cactusholder (Autodesk Fusion 360 design; units mm, degrees)
Autodesk Fusion 360 part; units mm, degrees
sketch "Sketch1" plane through (0, 0, 0) normal (0, 0, 1) x (1, 0, 0)
  circle A0 centre (0, 0) radius 37.5
  circle A1 centre (41.1956, 26.2031) radius 5
  spline S0 degree 5 poles (-34.1248, 15.5483) (-34.2892, 15.7362) (-35.0019, 16.448) (-36.6305, 17.4055) (-39.8225, 17.9751) (-44.8611, 17.5874) (-50.2206, 16.9014) (-53.5274, 17.4394) (-53.931, 20.0284) (-51.715, 24.3952) (-48.5491, 28.6137) (-45.8719, 31.6881) (-44.0593, 33.5751) (-43.1537, 34.4673) (-42.248, 35.3596) (-40.4379, 37.0417) (-37.7714, 39.1944) (-34.3544, 41.1861) (-30.0177, 42.3086) (-25.2467, 42.4584) (-19.8767, 42.1915) (-14.3394, 42.0733) (-9.6412, 42.5862) (-6.8287, 44.1058) (-6.6326, 46.8627) (-8.9316, 50.901) (-12.8621, 56.0874) (-17.1953, 62.1454) (-20.6408, 68.6812) (-22.1573, 75.2143) (-21.315, 81.2026) (-18.4614, 86.0812) (-14.3516, 89.3377) (-9.8763, 90.5804) (-5.7587, 89.6084) (-2.2448, 86.4855) (0.7698, 81.4936) (3.5863, 75.0781) (6.5537, 67.7955) (9.9317, 60.2619) (13.7133, 53.098) (17.6284, 46.8897) (21.2595, 42.1594) (24.1244, 39.3337) (25.7694, 38.7132) (25.8652, 40.4391) (24.2804, 44.4695) (21.0963, 50.5852) (16.6263, 58.3912) (11.4444, 67.316) (6.3871, 76.6199) (2.6215, 85.3808) (1.4925, 92.5512) (3.913, 97.1332) (9.9257, 98.341) (18.0512, 95.7377) (24.9795, 89.4537) (29.7272, 80.3543) (32.2443, 69.7321) (33.2851, 59.1225) (33.8442, 50.0699) (34.6188, 43.9145) (35.8347, 41.571) (35.9801, 43.3109) (34.7458, 48.5018) (32.945, 55.9404) (31.743, 64.1457) (32.2446, 71.6462) (34.811, 77.3174) (38.9242, 80.5216) (43.6598, 80.997) (47.9856, 78.8101) (51.1845, 74.2838) (53.0377, 67.9308) (53.6508, 60.3705) (53.3602, 52.251) (52.6058, 44.1681) (51.8225, 36.5886) (51.3137, 29.7638) (51.1609, 23.6723) (51.294, 18.1189) (51.5407, 12.8106) (51.6852, 7.444) (51.5193, 1.7821) (50.9065, -4.2483) (49.7806, -10.5689) (48.1193, -17.0032) (45.9267, -23.316) (43.2121, -29.2593) (39.9704, -34.6139) (36.1601, -39.2362) (31.7251, -43.0467) (26.6192, -46.015) (20.8312, -48.1455) (14.4061, -49.4634) (7.4769, -49.9996) (0.2576, -49.781) (-6.9991, -48.8285) (-14.0334, -47.152) (-20.6155, -44.7462) (-26.5781, -41.5878) (-31.8565, -37.6283) (-36.5088, -32.7991) (-40.6476, -27.0683) (-44.3788, -20.4938) (-47.7478, -13.2723) (-50.6588, -5.8037) (-52.8614, 1.2845) (-53.7725, 7.0105) (-52.8643, 10.3419) (-49.9006, 10.7215) (-46.0385, 8.5959) (-42.6562, 6.0361) (-40.1398, 4.8256) (-38.4302, 4.739) (-37.463, 4.9762) (-37.1537, 5.0843) knots 0.92424106 0.92424106 0.92424106 0.92424106 0.92424106 0.92424106 0.92727273 0.93636364 0.94545455 0.95454545 0.96363636 0.97272727 0.98181818 0.99090909 1 1 1 1 1 1.00909091 1.01818182 1.02727273 1.03636364 1.04545455 1.05454545 1.06363636 1.07272727 1.08181818 1.09090909 1.1 1.10909091 1.11818182 1.12727273 1.13636364 1.14545455 1.15454545 1.16363636 1.17272727 1.18181818 1.19090909 1.2 1.20909091 1.21818182 1.22727273 1.23636364 1.24545455 1.25454545 1.26363636 1.27272727 1.28181818 1.29090909 1.3 1.30909091 1.31818182 1.32727273 1.33636364 1.34545455 1.35454545 1.36363636 1.37272727 1.38181818 1.39090909 1.4 1.40909091 1.41818182 1.42727273 1.43636364 1.44545455 1.45454545 1.46363636 1.47272727 1.48181818 1.49090909 1.5 1.50909091 1.51818182 1.52727273 1.53636364 1.54545455 1.55454545 1.56363636 1.57272727 1.58181818 1.59090909 1.6 1.60909091 1.61818182 1.62727273 1.63636364 1.64545455 1.65454545 1.66363636 1.67272727 1.68181818 1.69090909 1.7 1.70909091 1.71818182 1.72727273 1.73636364 1.74545455 1.75454545 1.76363636 1.77272727 1.78181818 1.79090909 1.8 1.80909091 1.81818182 1.82727273 1.83636364 1.84545455 1.85454545 1.86363636 1.87272727 1.88181818 1.89090909 1.89532426 1.89532426 1.89532426 1.89532426 1.89532426 1.89532426
  line L0 (-7.3434, 102.5838) -> (33.3677, 91.2056)
  line L1 (33.0957, 46.9755) -> (37.6313, 38.7289)
  line L2 (-66.8334, 13.1525) -> (-33.0994, 7.1805)
  point P0 (-43.1537, 34.4673)
  point P1 (-22.3254, 42.3028)
  point P2 (-7.1303, 45.1644)
  point P3 (-21.3901, 73.2949)
  point P4 (-9.7001, 90.0328)
  point P5 (7.9129, 64.8764)
  point P6 (25.0933, 39.2325)
  point P7 (8.3567, 73.1958)
  point P8 (13.0121, 96.8947)
  point P9 (35.3635, 42.8522)
  point P10 (32.2623, 68.1236)
  point P11 (46.237, 79.3102)
  point P12 (52.0051, 38.0677)
  point P13 (51.5891, 5.8246)
  point P14 (42.8522, -29.5389)
  point P15 (17.6817, -48.6768)
  point P16 (-25.3785, -42.0201)
  point P17 (-51.3919, -3.1571)
  point P18 (-49.9664, 10.1665)
  point P19 (-52.3626, 17.6483)
  dimension "d1" = 75
  dimension "d2" = 10
  constraint coincident A0.centre origin
  constraint coincident A0 S0.end
  constraint coincident A0 S0.start
  constraint midpoint P8 L0
  constraint midpoint P9 L1
  constraint midpoint P18 L2
  measures "d1" diameter of A0
  measures "d2" diameter of A1
extrude "Extrude1" add sketch "Sketch1" along normal blind 8 contours A0 S0
fillet "Fillet1" radius 2.5 1 edges at (36.0213, -10.4269, 8)
